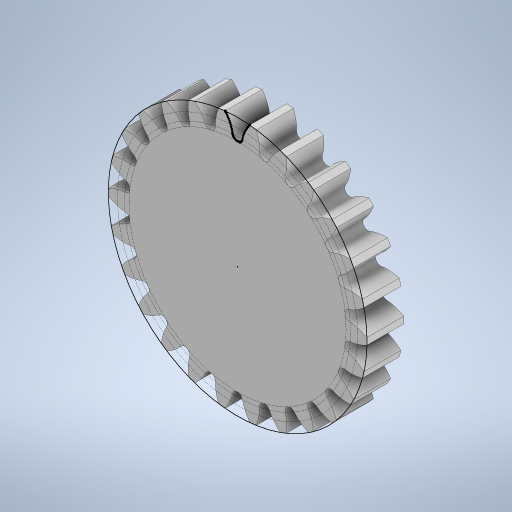
# Autodesk Inventor part: OnGiroGear
Saved by Autodesk Inventor 2024 (Build 280153000, 153)
## iProperties
Created: 2023-10-17
Part Number: OnGiroGear
Material: Generic
Document SubType Name: Modeling
Designer: Kippi
Density: 1 g/cm^3
Appearance: Default
Author: Kippi
Autodesk Inventor part; units mm, degrees
ref_plane "YZ Plane" through (0, 0, 0) normal (1, 0, 0) x (0, 1, 0)
ref_plane "XZ Plane" through (0, 0, 0) normal (0, 1, 0) x (-1, 0, 0)
ref_plane "XY Plane" through (0, 0, 0) normal (0, 0, 1) x (1, 0, 0)
sketch "Sketch1" plane through (0, 0, 0) normal (0, 0, 1) x (1, 0, 0)
  spline S0 degree 3 poles (-6.6381, 69.6845) (-6.4794, 69.4521) (-6.162, 68.9873) (-5.7096, 68.2742) (-5.2752, 67.5502) (-4.8623, 66.8136) (-4.472, 66.0648) (-4.1066, 65.3035) (-3.7689, 64.5296) (-3.4616, 63.7429) (-3.1927, 62.9426) (-2.958, 62.1304) (-2.8387, 61.4366) (-2.7173, 60.8868) (-2.5887, 60.4841) (-2.4199, 60.0967) (-2.2064, 59.7311) (-1.9798, 59.4605) (-1.7772, 59.2646) (-1.6078, 59.1384) (-1.4324, 59.02) (-1.241, 58.9304) (-1.0465, 58.8472) (-0.8409, 58.7976) (-0.6335, 58.7565) (-0.3516, 58.7459) (0, 58.7527) (0.3516, 58.7459) (0.6335, 58.7565) (0.8409, 58.7976) (1.0465, 58.8472) (1.241, 58.9304) (1.4324, 59.02) (1.6078, 59.1384) (1.7772, 59.2646) (1.9798, 59.4605) (2.2064, 59.7311) (2.4199, 60.0967) (2.5887, 60.4841) (2.7173, 60.8868) (2.8387, 61.4366) (2.958, 62.1304) (3.1927, 62.9426) (3.4616, 63.7429) (3.7689, 64.5296) (4.1066, 65.3035) (4.472, 66.0648) (4.8623, 66.8136) (5.2752, 67.5502) (5.7096, 68.2742) (6.162, 68.9873) (6.4794, 69.4521) (6.6381, 69.6845) knots 0 0 0 0 0.084428 0.168856 0.253284 0.337712 0.422139 0.506565 0.590991 0.675415 0.759837 0.844255 0.928666 0.970877 1.013073 1.05526 1.097443 1.139606 1.160716 1.181822 1.202924 1.224029 1.245128 1.266233 1.287336 1.308439 1.350654 1.392868 1.413971 1.435075 1.456179 1.477278 1.498383 1.519485 1.540591 1.561701 1.603865 1.646047 1.688235 1.730431 1.772641 1.857053 1.94147 2.025892 2.110316 2.194742 2.279168 2.363595 2.448023 2.532451 2.616879 2.701307 2.701307 2.701307 2.701307
  circle A0 centre (0, 0) radius 58.75 construction
  circle A1 centre (0, 0) radius 61.08 construction
  circle A2 centre (0, 0) radius 65 construction
  circle A3 centre (0, 0) radius 70
  point P0 (-6.1659, 68.9847)
  point P1 (-5.7126, 68.2724)
  point P2 (-5.2788, 67.5481)
  point P3 (-4.866, 66.8116)
  point P4 (-4.4761, 66.0627)
  point P5 (-4.1112, 65.3014)
  point P6 (-3.774, 64.5274)
  point P7 (-3.468, 63.7406)
  point P8 (-3.1984, 62.9406)
  point P9 (-2.9732, 62.127)
  point P10 (-2.8062, 61.2996)
  point P11 (-2.711, 60.8883)
  point P12 (-2.582, 60.4866)
  point P13 (-2.4125, 60.1003)
  point P14 (-2.1967, 59.7378)
  point P15 (-1.9275, 59.4133)
  point P16 (-1.7743, 59.268)
  point P17 (-1.6068, 59.1397)
  point P18 (-1.4297, 59.0248)
  point P19 (-1.2404, 58.9315)
  point P20 (-1.0447, 58.8528)
  point P21 (-0.8406, 58.799)
  point P22 (-0.6328, 58.7621)
  point P23 (-0.4221, 58.7499)
  point P24 (0, 58.75)
  point P25 (0.4221, 58.7499)
  point P26 (0.6328, 58.7621)
  point P27 (0.8406, 58.799)
  point P28 (1.0447, 58.8528)
  point P29 (1.2404, 58.9315)
  point P30 (1.4297, 59.0248)
  point P31 (1.6068, 59.1397)
  point P32 (1.7743, 59.268)
  point P33 (1.9275, 59.4133)
  point P34 (2.1967, 59.7378)
  point P35 (2.4125, 60.1003)
  point P36 (2.582, 60.4866)
  point P37 (2.711, 60.8883)
  point P38 (2.8062, 61.2996)
  point P39 (2.9732, 62.127)
  point P40 (3.1984, 62.9406)
  point P41 (3.468, 63.7406)
  point P42 (3.774, 64.5274)
  point P43 (4.1112, 65.3014)
  point P44 (4.4761, 66.0627)
  point P45 (4.866, 66.8116)
  point P46 (5.2788, 67.5481)
  point P47 (5.7126, 68.2724)
  point P48 (6.1659, 68.9847)
  constraints: 4 centre point, 2 point on circle, 107 other
extrude "Extrusion1" add sketch "Sketch1" against normal blind 20
extrude "Extrusion2" cut sketch "Sketch1" against normal blind 30 contours A3 S0 picked at (-0.8376, 66.9844)
pattern_circular "Circular Pattern1" count 26 over 360 about axis through (0, 0, 0) along (0, 0, -1) of "Extrusion2"
equation "\"d0\" = FaceWidth"
equation "\"Module\" = 5"
equation "\"PressureAngle\" = 20deg"
equation "\"UnitProfileClearance\" = 0.25"
equation "\"UnitRoundRadius\" = 0.35"
equation "\"RootDiameter\" = 117.5"
equation "\"BaseDiameter\" = 122.16004"
equation "\"FaceWidth\" = 20"
equation "\"HelixAngle\" = 0"
equation "\"UnitCorrection\" = 0"
equation "\"UnitAddendumModification\" = 0"
equation "\"CircularPitch\" = 15.707963"
equation "\"UnitBacklashShift\" = 0"
equation "\"TotalToolShift\" = 0"
equation "\"IsInternal\" = 0"
body "Solid1"
